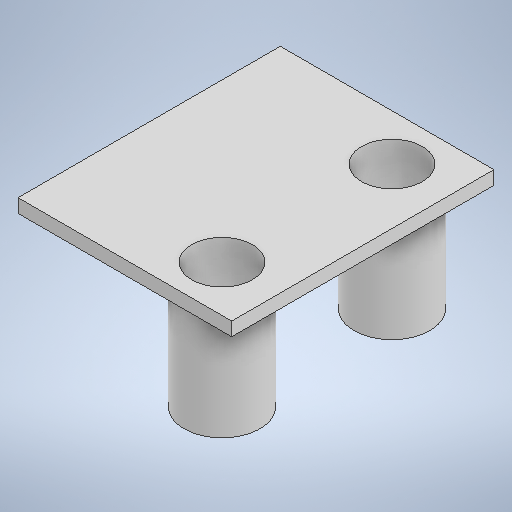
# Autodesk Inventor part: Крышка для клеммы
Saved by Autodesk Inventor 2025 (Build 290162000, 162)
## iProperties
Created: 2025-08-23
Part Number: Крышка для клеммы
Material: Типовые
Document SubType Name: Modeling
Designer: Makusimu
Density: 1 g/cm^3
Appearance: По умолчанию
Author: Makusimu
Autodesk Inventor part; units mm, degrees
ref_plane "YZ Plane" through (0, 0, 0) normal (1, 0, 0) x (0, 1, 0)
ref_plane "XZ Plane" through (0, 0, 0) normal (0, 1, 0) x (-1, 0, 0)
ref_plane "XY Plane" through (0, 0, 0) normal (0, 0, 1) x (1, 0, 0)
sketch "Эскиз1" plane through (0, 0, 0) normal (0, 1, 0) x (-1, 0, 0)
  line L0 (0, 0) -> (22, 0)
  line L1 (22, 0) -> (22, -27)
  line L2 (22, -27) -> (0, -27)
  line L3 (0, -27) -> (0, 0)
  dimension "d0" = 22
  dimension "d1" = 27
  constraints: 8 end point, 2 parallel, 1 horizontal, 1 perpendicular
  measures "d0" distance of L1.end L2.end
  measures "d1" distance of L0.end L1.end
extrude "Выдавливание1" add sketch "Эскиз1" along normal blind 1.4
sketch "Эскиз2" plane through (0, 0, 0) normal (0, -1, 0) x (1, 0, 0)
  circle A0 centre (-5.75, -4.75) radius 3.9
  circle A1 centre (-5.75, -22.25) radius 3.9
  line L0 (-22, 0) -> (0, 0) projected
  line L1 (0, 0) -> (0, -27) projected
  line L2 (0, -27) -> (-22, -27) projected
  dimension "d4" = 7.8
  dimension "d5" = 7.8
  dimension "d6" = 4.75
  dimension "d7" = 5.75
  dimension "d8" = 5.75
  dimension "d9" = 4.75
  constraints: 2 centre point
  measures "d4" diameter of A0
  measures "d5" diameter of A1
  measures "d6" distance from line of L0 A0.centre
  measures "d7" distance from line of L1 A0.centre
  measures "d8" distance from line of L1 A1.centre
  measures "d9" distance from line of L2 A1.centre
extrude "Выдавливание2" add sketch "Эскиз2" along normal blind 11.5
sketch "Эскиз3" plane through (-5.75, -11.5, -22.25) normal (0, -1, 0) x (1, 0, 0)
  circle A0 centre (0, 0) radius 2.75
  point P0 (5.75, 22.25)
  dimension "d12" = 5.5
  constraints: 1 centre point
  measures "d12" diameter of A0
extrude "Выдавливание3" cut sketch "Эскиз3" against normal blind 3
sketch "Эскиз4" plane through (-5.75, -11.5, -4.75) normal (0, -1, 0) x (1, 0, 0)
  circle A0 centre (0, 0) radius 2.75
  point P0 (5.75, 4.75)
  dimension "d13" = 5.5
  constraints: 1 centre point
  measures "d13" diameter of A0
extrude "Выдавливание4" cut sketch "Эскиз4" against normal blind 3
sketch "Эскиз5" plane through (0, 1.4, 0) normal (0, 1, 0) x (1, 0, 0)
  circle A0 centre (-5.75, 4.75) radius 3.9 projected
  circle A1 centre (-5.75, 4.75) radius 1.75
  circle A2 centre (-5.75, 22.2717) radius 1.75
  point P0 (0, 0)
  dimension "d20" = 3.5
  dimension "d21" = 3.5
  constraints: 2 centre point, 1 coincident
  measures "d20" diameter of A1
  measures "d21" diameter of A2
extrude "Выдавливание5" cut sketch "Эскиз5" against normal blind 11.5 contours A1 | A2
sketch "Эскиз6" plane through (0, 1.4, 0) normal (0, 1, 0) x (1, 0, 0)
  circle A0 centre (-5.75, 4.75) radius 2.75 projected
  circle A1 centre (-5.75, 4.75) radius 3.125
  circle A2 centre (-5.75, 22.25) radius 2.75 projected
  circle A3 centre (-5.75, 22.25) radius 3.125
  point P0 (0, 0)
  dimension "d24" = 6.25
  dimension "d25" = 6.25
  constraints: 2 centre point, 2 coincident
  measures "d24" diameter of A1
  measures "d25" diameter of A3
extrude "Выдавливание6" cut sketch "Эскиз6" against normal blind 6.3 contours A0 | A1 | A2 | A3
